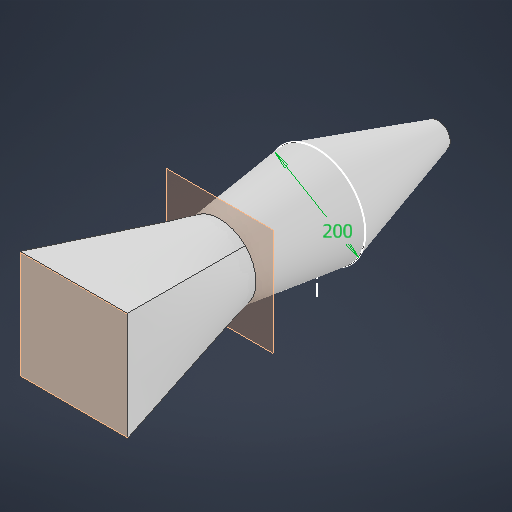
# Autodesk Inventor part: PartOne
Saved by Autodesk Inventor 2026 (Build 300175050, 175E)
## iProperties
Created: 2025-05-23
Part Number: PartOne
Material: Generic
Document SubType Name: Modeling
Designer: deniatmojoo
Density: 1 g/cm^3
Appearance: Default
Author: deniatmojoo
Autodesk Inventor part; units mm, degrees
ref_plane "YZ Plane" through (0, 0, 0) normal (1, 0, 0) x (0, 1, 0)
ref_plane "XZ Plane" through (0, 0, 0) normal (0, 1, 0) x (-1, 0, 0)
sketch "Sketch1" plane through (0, 0, 0) normal (0, 0, 1) x (1, 0, 0)
  circle A0 centre (0, 0) radius 25
  dimension "d0" = 50
  constraints: 1 centre point, 1 coincident
  measures "d0" diameter of A0
ref_plane "Work Plane1" through (0, 0, 250) normal (0, 0, 1) x (1, 0, 0)
sketch "Sketch2" plane through (0, 0, 250) normal (0, 0, 1) x (1, 0, 0)
  circle A0 centre (0, 0) radius 100
  line L0 (0, 0) -> (0, -169.491589)
  line L1 (-100, 0) -> (-100, -163.22364)
  dimension "d2" = 200
  constraints: 4 end point, 2 vertical, 1 coincident, 1 horizontal alignment, 2 other
sketch "Sketch1 outline for Loft1" plane through (0, 0, 0) normal (0, 0, 1) x (1, 0, 0)
  circle A0 centre (0, 0) radius 25
sketch "Sketch2 outline for Loft1" plane through (0, 0, 250) normal (0, 0, 1) x (1, 0, 0)
  circle A0 centre (0, 0) radius 100
loft "Loft1" add profiles "Sketch1 outline for Loft1", "Sketch2 outline for Loft1"
ref_plane "Work Plane6" through (0, 0, 450) normal (0, 0, 1) x (1, 0, 0)
sketch "Sketch7" plane through (0, 0, 450) normal (0, 0, 1) x (1, 0, 0)
  circle A0 centre (0, 0) radius 75
  dimension "d15" = 150
  constraints: 1 centre point, 1 coincident
  measures "d15" diameter of A0
sketch "Sketch7 outline for Loft2" plane through (0, 0, 450) normal (0, 0, 1) x (1, 0, 0)
  circle A0 centre (0, 0) radius 75
loft "Loft2" add profiles "Sketch7 outline for Loft2" section 1 edges at (-100, 0, 250)
ref_plane "Work Plane7" through (0, 0, 750) normal (0, 0, 1) x (1, 0, 0)
sketch "Sketch8" plane through (0, 0, 750) normal (0, 0, 1) x (1, 0, 0)
  line L0 (110.354309, -111.480379) -> (-110.354309, -111.480379)
  line L1 (-110.354309, -111.480379) -> (-110.354309, 111.480379)
  line L2 (-110.354309, 111.480379) -> (110.354309, 111.480379)
  line L3 (110.354309, 111.480379) -> (110.354309, -111.480379)
  line L4 (110.354309, -111.480379) -> (-110.354309, 111.480379) construction
  line L5 (-110.354309, -111.480379) -> (110.354309, 111.480379) construction
  point P0 (0, 0)
  constraints: 12 end point, 2 midpoint, 2 parallel, 1 horizontal, 1 perpendicular
sketch "Sketch8 outline for Loft3" plane through (0, 0, 750) normal (0, 0, 1) x (1, 0, 0)
  line L0 (110.354309, -111.480379) -> (-110.354309, -111.480379)
  line L1 (-110.354309, -111.480379) -> (-110.354309, 111.480379)
  line L2 (-110.354309, 111.480379) -> (110.354309, 111.480379)
  line L3 (110.354309, 111.480379) -> (110.354309, -111.480379)
loft "Loft3" add profiles "Sketch8 outline for Loft3" section 1 edges at (-75, 0, 450)
body "Solid1"
